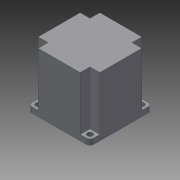
# Autodesk Inventor part: Stepper_Motor_Large
Saved by Autodesk Inventor 2015 (Build 190159000, 159)
## iProperties
Created: 2014-12-25
Part Number: Stepper_Motor_Large
Material: Generic
Document SubType Name: Modeling
Designer: Drew
Density: 1 g/cm^3
Appearance: Default
Author: Drew
Autodesk Inventor part; units mm, degrees
ref_plane "YZ Plane" through (0, 0, 0) normal (1, 0, 0) x (0, 1, 0)
ref_plane "XZ Plane" through (0, 0, 0) normal (0, 1, 0) x (-1, 0, 0)
ref_plane "XY Plane" through (0, 0, 0) normal (0, 0, 1) x (1, 0, 0)
sketch "Sketch1" plane through (0, 0, 0) normal (0, 1, 0) x (-1, 0, 0)
  line L0 (-28.2, -28.2) -> (28.2, -28.2)
  line L1 (28.2, -28.2) -> (28.2, 28.2)
  line L2 (28.2, 28.2) -> (-28.2, 28.2)
  line L3 (-28.2, 28.2) -> (-28.2, -28.2)
  line L4 (-28.2, -28.2) -> (28.2, 28.2) construction
  line L5 (28.2, -28.2) -> (-28.2, 28.2) construction
  line L6 (28.2, 28.2) -> (19.2, 28.2)
  line L7 (19.2, 28.2) -> (19.2, 19.2)
  line L8 (19.2, 19.2) -> (28.2, 19.2)
  line L9 (28.2, 19.2) -> (28.2, 28.2)
  line L10 (15.7012, 0) -> (-14.7312, 0)
  line L11 (0, 21.5613) -> (0, -24.5212)
  line L12 (28.2, -28.2) -> (19.2, -28.2)
  line L13 (19.2, -28.2) -> (19.2, -19.2)
  line L14 (19.2, -19.2) -> (28.2, -19.2)
  line L15 (28.2, -19.2) -> (28.2, -28.2)
  line L16 (-28.2, 28.2) -> (-19.2, 28.2)
  line L17 (-19.2, 28.2) -> (-19.2, 19.2)
  line L18 (-19.2, 19.2) -> (-28.2, 19.2)
  line L19 (-28.2, 19.2) -> (-28.2, 28.2)
  line L20 (-28.2, -28.2) -> (-19.2, -28.2)
  line L21 (-19.2, -28.2) -> (-19.2, -19.2)
  line L22 (-19.2, -19.2) -> (-28.2, -19.2)
  line L23 (-28.2, -19.2) -> (-28.2, -28.2)
  circle A0 centre (23.57, 23.57) radius 2.5
  circle A1 centre (23.57, -23.57) radius 2.5
  circle A2 centre (-23.57, 23.57) radius 2.5
  circle A3 centre (-23.57, -23.57) radius 2.5
  point P0 (0, 0)
  point P1 (0, 0)
  point P2 (0, 0)
  dimension "d0" = 56.4
  dimension "d1" = 56.4
  dimension "d2" = 9
  dimension "d3" = 9
  dimension "d6" = 47.14
  dimension "d7" = 47.14
  dimension "d8" = 5
  constraints: 48 end point, 12 symmetric about line, 4 centre point, 4 midpoint, 4 parallel, 3 horizontal, 2 perpendicular, 2 point on line, 1 vertical, 3 other
  measures "d0" distance of L0.end L1.end
  measures "d1" distance of L1.end L2.end
  measures "d2" distance of L18.start L18.end
  measures "d3" distance of L17.start L18.start
  measures "d6" diameter of A0.centre L10
  measures "d7" diameter of A0.centre L11
  measures "d8" diameter of A0
extrude "Extrusion1" add sketch "Sketch1" along normal blind 54 contours L21 L22 L3 L18 L17 L2 L7 L8 L1 L14 L13 L0
extrude "Extrusion2" add sketch "Sketch1" along normal blind 5 contours L3 L22 L21 L0 | L13 L14 L1 L0 | L3 L2 L17 L18 | L8 L7 L2 L1
fillet "Fillet1" radius 3.175 4 edges at (-28.2, 2.5, 28.2) (-28.2, 2.5, -28.2) (28.2, 2.5, -28.2) (28.2, 2.5, 28.2)
sketch "Sketch2" plane through (0, 0, 0) normal (0, -1, 0) x (1, 0, 0)
  circle A0 centre (0, 0) radius 19.05
  dimension "d12" = 38.1
  constraints: 1 centre point, 1 coincident
  measures "d12" diameter of A0
extrude "Extrusion3" add sketch "Sketch2" along normal blind 1.6
sketch "Sketch3" plane through (0, 0, 0) normal (0, -1, 0) x (1, 0, 0)
  circle A0 centre (0, 0) radius 3.175
  dimension "d15" = 6.35
  constraints: 1 centre point, 1 coincident
  measures "d15" diameter of A0
extrude "Extrusion4" add sketch "Sketch3" along normal blind 21
equation "\"d1\" = d0"
equation "\"d3\" = d2"
equation "\"d7\" = d6"
body "Solid1"
